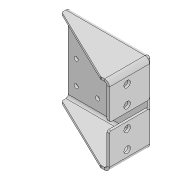
# Autodesk Inventor part: CCM_Mount_A
Saved by Autodesk Inventor 2020 (Build 240168000, 168)
## iProperties
Created: 2021-12-05
Part Number: CCM_Mount_A
Material: 一般
Document SubType Name: Sheet Metal
Designer: ken113
Density: 1 g/cm^3
Sheet Metal Rule: Default_mm
Appearance: 既定
Author: ken113
Autodesk Inventor part; units mm, degrees
note: some values were not read from the file. Chosen so that the rebuilt part matches the saved one: flange form of "プレート2".
ref_plane "YZ Plane" through (0, 0, 0) normal (1, 0, 0) x (0, 1, 0)
ref_plane "XZ Plane" through (0, 0, 0) normal (0, 1, 0) x (-1, 0, 0)
ref_plane "XY Plane" through (0, 0, 0) normal (0, 0, 1) x (1, 0, 0)
sketch "スケッチ1" plane through (0, 0, 0) normal (0, 0, 1) x (1, 0, 0)
  line L0 (-50, -50) -> (50, -50)
  line L1 (50, -50) -> (50, 50)
  line L2 (50, 50) -> (-50, 50)
  line L3 (-50, 50) -> (-50, -50)
  line L4 (-50, -50) -> (50, 50) construction
  line L5 (50, -50) -> (-50, 50) construction
  point P0 (0, 0)
  dimension "d0" = 100
  dimension "d1" = 100
  measures "d0" distance of L1.end L2.end
  measures "d1" distance of L2.end L0.start
extrude "プレート1" add sketch "スケッチ1" along normal blind 3
sketch "スケッチ2" plane through (-50, 47, 0) normal (0, 1, 0) x (-1, 0, 0)
  line L0 (-100, 0) -> (0, 0)
  line L1 (0, 0) -> (0, 57)
  line L2 (0, 57) -> (-100, 57)
  line L3 (-100, 57) -> (-100, 0)
  constraints: 6 end point, 1 horizontal, 1 perpendicular, 1 vertical
edge flange "フランジ1" height 57 angle 90 thickness 3 bend radius 3 thickness toward (0, 1, 0) relief tear relief width 3 relief depth 1.5 corner gap 3 corner form 0 edges at (0, 50, 3) (0, -50, 3) wall of the first edge with corners at (50, 47, 0) (-50, 47, 0) (-50, 47, 57) (50, 47, 57)
bend "曲げ1"
corner "コーナー1"
sketch "スケッチ3" plane through (53, 44, 57) normal (1, 0, 0) x (0, 1, 0)
  line L0 (0, -51) -> (0, 0)
  line L1 (0, 0) -> (-39, 0)
  line L2 (-39, 0) -> (-39, -51)
  line L3 (-39, -51) -> (0, -51)
  constraints: 6 end point, 1 horizontal, 1 perpendicular, 1 vertical
edge flange "フランジ2" height 45 angle 90 thickness 3 bend radius 3 thickness toward (1, 0, 0) relief tear relief width 3 relief depth 1.5 corner gap 3 corner form 0 edges at (50, 47, 31.5) (50, -47, 31.5) wall of the first edge with corners at (53, 44, 6) (53, 44, 57) (53, 5, 57) (53, 5, 6)
bend "曲げ2"
corner "コーナー2"
sketch "スケッチ4" plane through (-50, -50, 6) normal (0, -1, 0) x (1, 0, 0)
  line L0 (0, 0) -> (0, 51) projected
  line L1 (0, 5) -> (95, 51)
  line L2 (0, 51) -> (100, 51) projected
  line L3 (0, 0) -> (100, 0) projected
  line L4 (100, 51) -> (100, 0) projected
  point P0 (50, -6)
  dimension "d23" = 5
  dimension "d24" = 5
  constraints: 2 end point, 2 point on line
  measures "d23" distance from line of L1.start L3
  measures "d24" distance from line of L4 L1.end
extrude "押し出し1" cut sketch "スケッチ4" against normal through all contours L0 L2 L1
fillet "フィレット1" radius 2 8 edges at (-50, 48.5, 11) (-50, -48.5, 11) (45, 48.5, 57) (45, -48.5, 57) (54.5, 5, 57) (54.5, -5, 6) (54.5, 5, 6) (54.5, -5, 57)
sketch "スケッチ5" plane through (0, 0, 3) normal (0, 0, 1) x (1, 0, 0)
  line L0 (-40, -30) -> (-13, -30)
  line L1 (-13, -30) -> (-13, 30)
  line L2 (-13, 30) -> (-40, 30)
  line L3 (-40, 30) -> (-40, -30)
  line L4 (-40, -30) -> (-13, 30) construction
  line L5 (-13, -30) -> (-40, 30) construction
  line L6 (-50, -44) -> (-50, 44) projected
  point P0 (0, 0)
  point P1 (-26.5, 0)
  point P2 (-26.5, 0)
  point P3 (-40, 0)
  point P4 (-13, 0)
  dimension "d28" = 27
  dimension "d29" = 10
  dimension "d30" = 60
  constraints: 12 end point, 5 midpoint, 2 parallel, 1 horizontal, 1 horizontal alignment, 1 perpendicular
  measures "d28" distance of L1.end L2.end
  measures "d29" distance between parallel lines of L3 L6
  measures "d30" distance of L2.end L0.start
hole "穴1" at (-40, 0, 3) at (-13, 0, 3) at (-40, -30, 3) at (-40, 30, 3) at (-13, -30, 3) at (-13, 30, 3) direction (0, 0, -1) diameter 5.2 end through all
sketch "スケッチ6" plane through (53, 44, 6) normal (-1, 0, 0) x (0, 0, 1)
  arc A0 (0, -37) -> (2, -39) centre (2, -37) ccw projected
  line L0 (2, -39) -> (49, -39) projected
  arc A1 (49, -39) -> (51, -37) centre (49, -37) ccw projected
  line L1 (51, -37) -> (51, 0) projected
  line L2 (51, 0) -> (0, 0) projected
  line L3 (0, -37) -> (0, 0) projected
  arc A2 (2, -49) -> (0, -51) centre (2, -51) ccw projected
  line L4 (0, -51) -> (0, -88) projected
  line L5 (0, -88) -> (51, -88) projected
  line L6 (51, -51) -> (51, -88) projected
  arc A3 (51, -51) -> (49, -49) centre (49, -51) ccw projected
  line L7 (49, -49) -> (2, -49) projected
  point P0 (-6, -44)
  point P1 (28.5, -8)
  point P2 (28.5, -31)
  point P3 (28.5, -57)
  point P4 (28.5, -80)
  dimension "d38" = 22.5
  dimension "d39" = 8
  dimension "d40" = 8
  dimension "d41" = 8
  dimension "d42" = 8
  constraints: 3 vertical alignment
  measures "d38" distance from line of point (28.5, -80) L6
  measures "d39" distance from line of point (28.5, -80) L5
  measures "d40" distance from line of L7 point (28.5, -57)
  measures "d41" distance from line of point (28.5, -31) L0
  measures "d42" distance from line of L2 point (28.5, -8)
hole "穴2" at (53, 36, 34.5) at (53, 13, 34.5) at (53, -13, 34.5) at (53, -36, 34.5) direction (1, 0, 0) diameter 8.2 end through all
equation "\"d36\" = Thickness"
equation "\"d48\" = Thickness"
equation "\"d2\" = Thickness"
equation "\"d3\" = BendReliefWidth"
equation "\"d4\" = BendReliefDepth"
equation "\"d5\" = MinimumRemnant"
equation "\"d6\" = TransitionRadius"
equation "\"d9\" = BendRadius"
equation "\"d10\" = CornerReliefSize"
equation "\"d11\" = GapSize"
equation "\"d12\" = JacobiRadiusSize"
equation "\"d13\" = BendReliefWidth"
equation "\"d14\" = BendReliefDepth"
equation "\"d15\" = MinimumRemnant"
equation "\"d16\" = TransitionRadius"
equation "\"d19\" = BendRadius"
equation "\"d20\" = CornerReliefSize"
equation "\"d21\" = GapSize"
equation "\"d22\" = JacobiRadiusSize"
equation "\"BendRadius\" = Thickness"
equation "\"BendReliefWidth\" = Thickness"
equation "\"BendReliefDepth\" = 0.5 * Thickness"
equation "\"CornerReliefSize\" = 4 * Thickness"
equation "\"MinimumRemnant\" = 2 * Thickness"
equation "\"TransitionRadius\" = BendRadius"
equation "\"JacobiRadiusSize\" = BendRadius"
equation "\"GapSize\" = Thickness"
equation "\"Thickness\" = 3"
